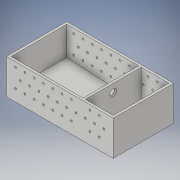
# Autodesk Inventor part: bottomA
Saved by Autodesk Inventor 2019 (Build 230136000, 136)
## iProperties
Created: 2018-07-24
Part Number: bottomA
Material: Generic
Document SubType Name: Modeling
Designer: email
Density: 1 g/cm^3
Appearance: Default
Author: email
Autodesk Inventor part; units mm, degrees
ref_plane "YZ Plane" through (0, 0, 0) normal (1, 0, 0) x (0, 1, 0)
ref_plane "XZ Plane" through (0, 0, 0) normal (0, 1, 0) x (-1, 0, 0)
ref_plane "XY Plane" through (0, 0, 0) normal (0, 0, 1) x (1, 0, 0)
sketch "Sketch1" plane through (0, 0, 0) normal (0, 1, 0) x (-1, 0, 0)
  line L0 (0, 0) -> (230, 0)
  line L1 (230, 0) -> (230, -130)
  line L2 (230, -130) -> (0, -130)
  line L3 (0, -130) -> (0, 0)
  dimension "d0" = 130
  dimension "d1" = 230
  constraints: 8 end point, 2 parallel, 1 horizontal, 1 perpendicular
  measures "d0" distance of L2.end L0.start
  measures "d1" distance of L1.end L2.end
extrude "Extrusion1" add sketch "Sketch1" along normal blind 5
sketch "Sketch2" plane through (0, 5, 0) normal (0, 1, 0) x (1, 0, 0)
  line L0 (-230, 130) -> (-230, 0) projected
  line L1 (0, 0) -> (0, 130) projected
  line L2 (-230, 0) -> (0, 0)
  line L3 (0, 0) -> (0, 130)
  line L4 (0, 130) -> (-230, 130)
  line L5 (-230, 130) -> (-230, 0)
  line L6 (-225, 5) -> (-5, 5)
  line L7 (-5, 5) -> (-5, 125)
  line L8 (-5, 125) -> (-225, 125)
  line L9 (-225, 125) -> (-225, 5)
  dimension "d4" = 5
  dimension "d6" = 5
  dimension "d7" = 5
  dimension "d8" = 5
  constraints: 16 end point, 4 parallel, 2 horizontal, 2 perpendicular
  measures "d4" distance between parallel lines of L4 L8
  measures "d6" distance between parallel lines of L2 L6
  measures "d7" distance between parallel lines of L1 L7
  measures "d8" distance between parallel lines of L0 L9
extrude "Extrusion2" add sketch "Sketch2" along normal blind 70
sketch "Sketch3" plane through (0, 5, 0) normal (0, 1, 0) x (1, 0, 0)
  line L0 (-225, 5) -> (-5, 5) projected
  line L1 (-5, 125) -> (-225, 125) projected
  line L2 (-65, 5) -> (-70, 5)
  line L3 (-70, 5) -> (-70, 125)
  line L4 (-70, 125) -> (-65, 125)
  line L5 (-65, 125) -> (-65, 5)
  line L6 (-5, 125) -> (-5, 5) projected
  point P0 (0, 0)
  dimension "d11" = 5
  dimension "d12" = 60
  constraints: 8 end point, 2 parallel, 2 point on line, 1 horizontal, 1 perpendicular
  measures "d11" distance between parallel lines of L5 L3
  measures "d12" distance between parallel lines of L5 L6
extrude "Extrusion3" add sketch "Sketch3" along normal up to surface (70 mm away) contours L3 L1 L5 L0
sketch "Sketch4" plane through (-65, 5, -5) normal (1, 0, 0) x (0, 0, -1)
  circle A0 centre (60, 52.5) radius 7.5
  line L0 (120, 70) -> (0, 70) projected
  point P0 (-5, -5)
  point P1 (60, 70)
  point P2 (60, 70)
  point P3 (60, 70)
  dimension "d15" = 15
  dimension "d16" = 17.5
  constraints: 3 midpoint, 1 centre point, 1 coincident, 1 vertical alignment
  measures "d15" diameter of A0
  measures "d16" distance from line of A0.centre L0
extrude "Extrusion4" cut sketch "Sketch4" against normal up to surface (5 mm away)
sketch "Sketch6" plane through (-225, 5, -125) normal (0, 0, 1) x (1, 0, 0)
  line L0 (155, 0) -> (0, 0) projected
  line L1 (0, 0) -> (155, 0)
  line L2 (155, 0) -> (0, 8.1232)
  line L3 (0, 0) -> (0, 70) projected
  line L4 (0, 8.1232) -> (0, 0)
  line L5 (160, 0) -> (220, 5.2493)
  line L6 (220, 0) -> (220, 70) projected
  line L7 (220, 5.2493) -> (220, 0)
  line L8 (220, 0) -> (160, 0)
  point P0 (225, -5)
  dimension "d38" = 5
  dimension "d39" = 3
  constraints: 12 end point, 3 collinear, 2 point on line, 1 perpendicular
  measures "d38" angle of L8 L5
  measures "d39" angle of L0 L2
extrude "Extrusion5" add sketch "Sketch6" along normal up to surface (120 mm away)
sketch "Sketch7" plane through (0, 75, 0) normal (0, 1, 0) x (1, 0, 0)
  line L0 (-225, 125) -> (-70, 125) projected
  line L1 (-70, 5) -> (-225, 5) projected
  line L2 (-70, 125) -> (-73, 125)
  line L3 (-73, 125) -> (-73, 5)
  line L4 (-73, 5) -> (-70, 5)
  line L5 (-70, 5) -> (-70, 125)
  line L6 (-65, 125) -> (-65, 5) projected
  line L7 (-65, 125) -> (-62, 125)
  line L8 (-62, 125) -> (-62, 5)
  line L9 (-62, 5) -> (-65, 5)
  line L10 (-65, 5) -> (-65, 125)
  point P0 (0, 0)
  point P1 (-71.5, 5)
  point P2 (-63.5, 5)
  dimension "d42" = 3
  dimension "d43" = 3
  constraints: 16 end point, 4 parallel, 2 horizontal, 2 midpoint, 2 perpendicular, 1 horizontal alignment, 1 point on line
  measures "d42" distance between parallel lines of L5 L3
  measures "d43" distance between parallel lines of L6 L8
extrude "Extrusion6" cut sketch "Sketch7" against normal through all
sketch "Sketch8" plane through (0, 0, 0) normal (0, -1, 0) x (1, 0, 0)
  line L0 (-230, -130) -> (0, -130) projected
  line L1 (-230, 0) -> (-230, -130) projected
  line L2 (-230, -130) -> (-230, 0) projected
  line L3 (-230, -65) -> (0, -65)
  line L4 (0, -130) -> (0, 0) projected
  line L5 (-115, -130) -> (-115, 0)
  point P0 (-210, -115)
  point P1 (-210, -15)
  point P2 (-20, -115)
  point P3 (-20, -15)
  dimension "d46" = 15
  dimension "d47" = 20
  constraints: 4 end point, 3 midpoint, 3 symmetric about line, 1 vertical
  measures "d46" distance from line of L0 point (-210, -115)
  measures "d47" distance from line of point (-210, -115) L1
hole "Hole2" at (-210, 0, -115) at (-210, 0, -15) at (-20, 0, -15) at (-20, 0, -115) direction (0, 1, 0) diameter 4 depth 7.5
sketch "Sketch9" plane through (-230, 0, 0) normal (0, 0, 1) x (1, 0, 0)
  line L0 (20, 65) -> (233.5105, 65)
  line L1 (20, 45) -> (233.5105, 45)
  line L2 (234.6135, 25) -> (20, 25)
  line L3 (0, 75) -> (230, 75) projected
  line L4 (0, 0) -> (0, 75) projected
  point P0 (230, 0)
  point P1 (30, 45)
  point P2 (40, 65)
  point P3 (50, 45)
  point P4 (40, 25)
  point P5 (60, 65)
  point P6 (70, 45)
  point P7 (60, 25)
  point P8 (80, 65)
  point P9 (90, 45)
  point P10 (80, 25)
  point P11 (100, 65)
  point P12 (110, 45)
  point P13 (100, 25)
  point P14 (120, 65)
  point P15 (130, 45)
  point P16 (120, 25)
  point P17 (140, 65)
  point P18 (150, 45)
  point P19 (140, 25)
  point P20 (170, 45)
  point P21 (180, 65)
  point P22 (190, 45)
  point P23 (180, 25)
  point P24 (200, 65)
  point P25 (210, 45)
  point P26 (200, 25)
  dimension "d55" = 20
  dimension "d56" = 20
  dimension "d57" = 10
  dimension "d58" = 20
  dimension "d59" = 10
  dimension "d62" = 20
  constraints: 6 end point, 4 horizontal, 2 coincident, 2 vertical alignment, 1 point on line, 23 other
  measures "d55" distance between parallel lines of L1 L0
  measures "d56" distance between parallel lines of L2 L1
  measures "d57" distance between parallel lines of L3 L0
  measures "d58" distance from line of L4 L0.start
  measures "d59" horizontal distance of point (30, 45) point (20, 65)
  measures "d62" distance of point (20, 65) point (40, 65)
hole "Hole3" at (-210, 65, 0) at (-200, 45, 0) at (-210, 25, 0) at (-190, 65, 0) at (-180, 45, 0) at (-190, 25, 0) at (-170, 65, 0) at (-160, 45, 0) at (-170, 25, 0) at (-150, 65, 0) at (-140, 45, 0) at (-150, 25, 0) at (-130, 65, 0) at (-120, 45, 0) at (-130, 25, 0) at (-110, 65, 0) at (-100, 45, 0) at (-110, 25, 0) at (-90, 65, 0) at (-80, 45, 0) at (-90, 25, 0) at (-50, 65, 0) at (-40, 45, 0) at (-50, 25, 0) at (-30, 65, 0) at (-20, 45, 0) at (-30, 25, 0) at (-60, 45, 0) direction (0, 0, -1) diameter 4 end through all
equation "\"d4\" = d8"
equation "\"d6\" = d7"
equation "\"d7\" = d8"
equation "\"d43\" = d42"
body "Solid1"
